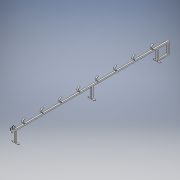
# Autodesk Inventor part: Stand
Saved by Autodesk Inventor 2017 (Build 210142000, 142)
## iProperties
Created: 2017-10-30
Part Number: Stand
Material: Generic
Document SubType Name: Modeling
Designer: DesignPC02
Density: 1 g/cm^3
Appearance: Default
Author: DesignPC02
Autodesk Inventor part; units mm, degrees
ref_plane "YZ Plane" through (0, 0, 0) normal (1, 0, 0) x (0, 1, 0)
ref_plane "XZ Plane" through (0, 0, 0) normal (0, 1, 0) x (-1, 0, 0)
ref_plane "XY Plane" through (0, 0, 0) normal (0, 0, 1) x (1, 0, 0)
sketch "Sketch1" plane through (0, 0, 0) normal (0, 0, 1) x (1, 0, 0)
  line L0 (0, 0) -> (25, 0)
  line L1 (25, 0) -> (25, 2900)
  line L2 (25, 2900) -> (0, 2900)
  line L3 (0, 2900) -> (0, 0)
  dimension "d0" = 25
  dimension "d1" = 2900
  constraints: 8 end point, 2 parallel, 1 horizontal, 1 perpendicular
  measures "d0" distance of L2.end L1.end
  measures "d1" distance of L1.end L0.end
extrude "Extrusion1" add sketch "Sketch1" along normal blind 25
sketch "Sketch2" plane through (0, 0, 0) normal (0, 0, -1) x (-1, 0, 0)
  line L0 (-25, 0) -> (-25, 2900) projected
  line L1 (0, 2900) -> (0, 0) projected
  line L2 (-25, 2900) -> (0, 2900)
  line L3 (0, 2900) -> (0, 2875)
  line L4 (0, 2875) -> (-25, 2875)
  line L5 (-25, 2875) -> (-25, 2900)
  dimension "d4" = 25
  constraints: 8 end point, 2 parallel, 1 horizontal, 1 perpendicular, 1 point on line
  measures "d4" distance of L2.end L3.end
extrude "Extrusion2" add sketch "Sketch2" along normal blind 200
sketch "Sketch3" plane through (0, 2875, 0) normal (0, -1, 0) x (1, 0, 0)
  line L0 (0, -200) -> (0, 25) projected
  line L1 (25, -200) -> (25, 25) projected
  line L2 (0, -200) -> (25, -200)
  line L3 (25, -200) -> (25, -175)
  line L4 (25, -175) -> (0, -175)
  line L5 (0, -175) -> (0, -200)
  point P0 (0, 0)
  dimension "d7" = 25
  constraints: 8 end point, 2 parallel, 1 horizontal, 1 perpendicular, 1 point on line
  measures "d7" distance of L3.end L2.end
extrude "Extrusion3" add sketch "Sketch3" along normal blind 200
sketch "Sketch4" plane through (0, 2875, -175) normal (0, 0, 1) x (1, 0, 0)
  line L0 (25, -200) -> (0, -200) projected
  line L1 (25, 25) -> (25, -200) projected
  line L2 (0, -200) -> (25, -200)
  line L3 (25, -200) -> (25, -175)
  line L4 (25, -175) -> (0, -175)
  line L5 (0, -175) -> (0, -200)
  point P0 (0, -2875)
  dimension "d10" = 25
  constraints: 8 end point, 2 parallel, 1 horizontal, 1 perpendicular, 1 point on line
  measures "d10" distance of L3.end L2.end
extrude "Extrusion4" add sketch "Sketch4" along normal up to next
sketch "Sketch6" plane through (0, 0, 25) normal (-1, 0, 0) x (0, 0, 1)
  line L0 (-225, 2900) -> (-225, 2675) projected
  line L1 (-225, 2675) -> (-220, 2675)
  line L2 (-220, 2675) -> (-220, 2700)
  line L3 (-220, 2700) -> (-225, 2700)
  line L4 (-225, 2700) -> (-225, 2675)
  point P0 (-25, 0)
  dimension "d13" = 5
  dimension "d14" = 25
  constraints: 8 end point, 2 parallel, 1 horizontal, 1 perpendicular
  measures "d13" distance of L3.end L2.end
  measures "d14" distance of L2.end L1.end
extrude "Extrusion5" add sketch "Sketch6" along normal blind 50 and the other way blind 75
pattern_linear "Rectangular Pattern1" count 3 spacing 1404 along (0, -1, 0) of "Extrusion2"
sketch "Sketch7" plane through (0, 0, 25) normal (-1, 0, 0) x (0, 0, 1)
  line L0 (-225, 1496) -> (-225, 1471) projected
  line L1 (-25, 1471) -> (-225, 1471) projected
  line L2 (-225, 1496) -> (-220, 1496)
  line L3 (-220, 1496) -> (-220, 1471)
  line L4 (-220, 1471) -> (-225, 1471)
  line L5 (-225, 1471) -> (-225, 1496)
  point P0 (-25, 0)
  dimension "d22" = 5
  constraints: 8 end point, 2 parallel, 1 horizontal, 1 perpendicular, 1 point on line
  measures "d22" distance of L3.end L4.end
extrude "Extrusion6" add sketch "Sketch7" along normal blind 50 and the other way blind 75
pattern_linear "Rectangular Pattern2" count 2 spacing 1404 along (0, -1, 0) of "Extrusion6"
sketch "Sketch8" plane through (0, 0, 25) normal (-1, 0, 0) x (0, 0, 1)
  arc A0 (-0.0707, 2610) -> (83.9293, 2610) centre (41.9293, 2610) ccw
  arc A1 (3.9293, 2610) -> (79.9293, 2610) centre (41.9293, 2610) ccw
  line L0 (-0.0707, 2610) -> (3.9293, 2610)
  line L1 (0, 0) -> (0, 2900) projected
  line L2 (79.9293, 2610) -> (83.9293, 2610)
  line L3 (0, 2900) -> (0, 0) projected
  line L4 (0, 2900) -> (42, 2900)
  point P0 (-25, 0)
  dimension "d31" = 4
  dimension "d39" = 42
  dimension "d40" = 290
  constraints: 6 end point, 4 point on circle, 2 centre point, 1 collinear, 1 horizontal, 1 perpendicular
  measures "d31" radial gap between concentric circles of A0 A1
  measures "d39" distance of L1.end L4.end
  measures "d40" distance of A0.centre L4.end
extrude "Extrusion7" add sketch "Sketch8" against normal up to surface (25 mm away)
pattern_linear "Rectangular Pattern3" count 8 spacing 338 along (0, -1, 0) of "Extrusion7"
sketch "Sketch10" plane through (0, 2900, -200) normal (-1, 0, 0) x (0, 0, 1)
  line L0 (200, -2900) -> (225, -2900) projected
  line L1 (225, -2900) -> (267, -2900)
  dimension "d41" = 42
  constraints: 2 end point, 1 horizontal
  measures "d41" distance of L0.end L1.end
body "Solid1"
